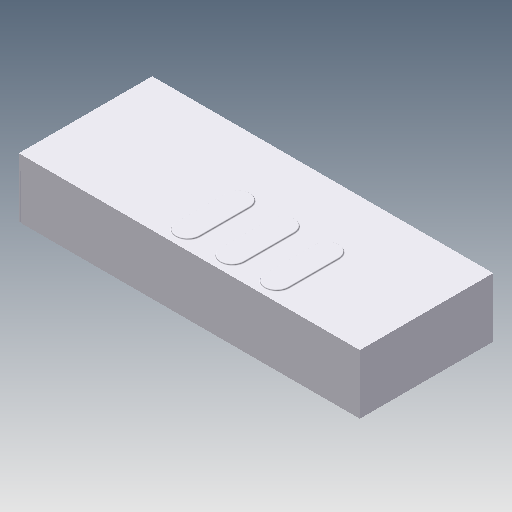
# Autodesk Inventor part: config - interface module
Saved by Autodesk Inventor 2020 (Build 240152000, 152)
## iProperties
Created: 2005-12-05
Part Number: config - interface module
Document SubType Name: Modeling
Designer: Simon.Ng@autodesk.com
Stock Number: config - interface module
Density: 1 g/cm^3
Material: Generic
Mass: 106.435 g
Surface Area: 212.581 cm^2
Volume: 106.435 cm^3
Appearance: Teflon
Company: Autodesk Asia Pte. Ltd.
Title: PC Demo
Author: Simon.Ng@autodesk.com
Autodesk Inventor part; units mm, degrees
ref_plane "YZ Plane" through (0, 0, 0) normal (1, 0, 0) x (0, 1, 0)
ref_plane "XZ Plane" through (0, 0, 0) normal (0, 1, 0) x (-1, 0, 0)
ref_plane "XY Plane" through (0, 0, 0) normal (0, 0, 1) x (1, 0, 0)
sketch "Sketch1" plane through (0, 0, 0) normal (0, 0, 1) x (1, 0, 0)
  line L0 (0, 26) -> (0, -2) projected
  line L1 (-69, 0) -> (92, 0) projected
  line L2 (-57.5, 0) -> (57.5, 0)
  line L3 (57.5, 0) -> (57.5, 20)
  line L4 (57.5, 20) -> (-57.5, 20)
  line L5 (-57.5, 20) -> (-57.5, 0)
  dimension "d0" = 115
  dimension "d1" = 20
  constraints: 8 end point, 2 parallel, 1 horizontal, 1 perpendicular, 1 point on line, 1 other
  measures "d0" distance of L3.end L4.end
  measures "d1" distance of L2.end L3.end
extrude "Extrusion1" add sketch "Sketch1" along normal blind 45
sketch "Sketch3" plane through (0, 0, 45) normal (0, 0, 1) x (1, 0, 0)
  line L0 (57.5, 0) -> (-57.5, 0) projected
  line L1 (57.5, 20) -> (57.5, 0) projected
  line L2 (57, 15) -> (56.8, 15)
  line L3 (56.8, 15) -> (56.8, 0)
  line L4 (56.8, 0) -> (57, 0)
  line L5 (57, 0) -> (57, 15)
  dimension "d8" = 0.5
  dimension "d9" = 0.2
  dimension "d10" = 15
  constraints: 8 end point, 2 parallel, 1 horizontal, 1 perpendicular, 1 point on line
  measures "d8" distance between parallel lines of L1 L5
  measures "d9" distance of L2.start L2.end
  measures "d10" distance of L2.end L3.end
extrude "Extrusion3" cut sketch "Sketch3" against normal blind 5
mirror "Mirror1" about plane through (0, 0, 0) normal (1, 0, 0) of "Extrusion3"
sketch "Sketch4" plane through (0, 0, 45) normal (0, 0, 1) x (1, 0, 0)
  line L0 (57.5, 20) -> (57.5, 0) construction
  line L1 (57, 15) -> (57.5, 15)
  constraints: 2 end point, 1 perpendicular, 1 point on line
split_face "Split1"
sketch "Sketch5" plane through (57.5, 0, 0) normal (1, 0, 0) x (0, 0, -1)
  line L0 (-45, 20) -> (-45, 15) construction
  line L1 (0, 20) -> (-45, 20) construction
  line L2 (-45, 15) -> (-25, 15)
  line L3 (-25, 15) -> (-15, 18)
  line L4 (-15, 18) -> (-15, 20)
  dimension "d13" = 30
  dimension "d14" = 2
  dimension "d15" = 20
  constraints: 6 end point, 1 parallel, 1 perpendicular, 1 point on line
  measures "d13" distance between parallel lines of L0 L4
  measures "d14" distance of L3.end L4.end
  measures "d15" distance of L0.end L2.end
split_face "Split2"
sketch "Sketch6" plane through (-57.5, 20, 0) normal (0, 1, 0) x (1, 0, 0)
  line L0 (0, -15) -> (0, -45) construction
  line L1 (115, -15) -> (0, -15)
  constraints: 2 end point, 1 perpendicular
split_face "Split3"
sketch "Sketch7" plane through (-57.5, 20, 45) normal (0, 1, 0) x (1, 0, 0)
  line L0 (0, 0) -> (115, 0) projected
  line L1 (115, 30) -> (115, 0) projected
  line L2 (77, 23) -> (85, 23)
  line L3 (85, 23) -> (85, 6)
  line L4 (85, 6) -> (77, 6)
  line L5 (77, 6) -> (77, 23)
  circle A0 centre (81, 23) radius 4
  circle A1 centre (81, 6) radius 4
  dimension "d16" = 25
  dimension "d17" = 8
  dimension "d18" = 30
  dimension "d19" = 6
  constraints: 8 end point, 2 horizontal alignment, 2 midpoint, 2 parallel, 1 horizontal, 1 perpendicular, 4 other
  measures "d17" distance between parallel lines of L5 L3
  measures "d18" distance between parallel lines of L1 L3
  measures "d19" distance between parallel lines of L0 L4
extrude "Extrusion4" add sketch "Sketch7" along normal blind 0.5
fillet "Fillet1" radius 0.25 8 edges at (23.5, 20, 43) (19.5, 20, 30.5) (23.5, 20, 18) (27.5, 20, 30.5) (23.5, 20.5, 43) (19.5, 20.5, 30.5) (23.5, 20.5, 18) (27.5, 20.5, 30.5)
pattern_linear "Rectangular Pattern1" count 3 spacing 15 along (-1, 0, 0) of "Extrusion4", "Fillet1"
sketch "Sketch8" plane through (-56.8, 0, 45) normal (0, -1, 0) x (1, 0, 0)
  line L0 (-0.7, -45) -> (114.3, -45) projected
  line L1 (114.3, -45) -> (114.3, 0) projected
  line L2 (0, -5) -> (-0.2, -5) projected
  line L3 (104.3, -10.1321) -> (104.3, -39.4486) construction
  line L4 (96.3, -15.2854) -> (96.3, -32.9211) construction
  circle A0 centre (104.3, -35) radius 3.5
  circle A1 centre (104.3, -35) radius 1.75
  circle A2 centre (104.3, -23) radius 3.5
  circle A3 centre (104.3, -23) radius 1.75
  circle A4 centre (104.3, -11) radius 3.5
  circle A5 centre (104.3, -11) radius 1.75
  circle A6 centre (96.3, -17) radius 1.75
  circle A7 centre (96.3, -17) radius 3.5
  circle A8 centre (96.3, -29) radius 1.75
  circle A9 centre (96.3, -29) radius 3.5
  dimension "d26" = 3.5
  dimension "d27" = 7
  dimension "d28" = 10
  dimension "d29" = 10
  dimension "d30" = 12
  dimension "d31" = 12
  dimension "d32" = 8
  dimension "d33" = 12
  dimension "d34" = 16
  constraints: 10 centre point, 8 equal radius, 5 coincident, 5 point on line, 4 end point, 1 parallel, 1 perpendicular
  measures "d26" diameter of A1
  measures "d27" diameter of A0
  measures "d28" distance between parallel lines of L1 L3
  measures "d29" distance from line of L0 A0.centre
  measures "d30" distance of A2.centre A0.centre
  measures "d31" distance of A2.centre A4.centre
  measures "d32" distance between parallel lines of L3 L4
  measures "d33" distance of A8.centre A6.centre
  measures "d34" distance from line of L0 A9.centre
extrude "Extrusion5" add sketch "Sketch8" along normal blind 5
sketch "Sketch9" plane through (-56.8, 0, 45) normal (0, -1, 0) x (1, 0, 0)
  line L0 (-0.7, -45) -> (114.3, -45) projected
  line L1 (114.3, -45) -> (114.3, 0) projected
  line L2 (0, -5) -> (-0.2, -5) projected
  circle A0 centre (79.3, -18) radius 6
  circle A1 centre (79.3, -33) radius 6
  line L3 (79.3, -18) -> (79.3, -33) construction
  dimension "d37" = 35
  dimension "d38" = 12
  dimension "d39" = 15
  dimension "d40" = 12
  constraints: 2 centre point, 2 end point, 1 equal radius, 1 perpendicular
  measures "d37" distance between parallel lines of L1 L3
  measures "d38" diameter of A1
  measures "d39" distance of L3.end L3.start
  measures "d40" distance from line of L0 L3.end
extrude "Extrusion6" add sketch "Sketch9" along normal blind 2
sketch "Sketch10" plane through (22.5, -2, 27) normal (0, -1, 0) x (1, 0, 0)
  circle A0 centre (0, 0) radius 6 projected
  line L0 (-4.0311, -2) -> (-2.5311, -2)
  line L1 (-2.5311, -2) -> (-2.5311, -3.7207)
  line L2 (4.0311, -2) -> (2.5311, -2)
  line L3 (2.5311, -2) -> (2.5311, -3.7207)
  line L4 (0, 0) -> (0, 4.5) construction
  line L5 (-1.5, 4.2426) -> (-1.5, 3.2426)
  line L6 (-1.5, 3.2426) -> (1.5, 3.2426)
  line L7 (1.5, 3.2426) -> (1.5, 4.2426)
  circle A1 centre (0, 0) radius 5
  arc A2 (-1.5, 4.2426) -> (-4.0311, -2) centre (0, 0) ccw
  arc A3 (-2.5311, -3.7207) -> (2.5311, -3.7207) centre (0, 0) ccw
  arc A4 (4.0311, -2) -> (1.5, 4.2426) centre (0, 0) ccw
  dimension "d44" = 2
  dimension "d45" = 1.5
  dimension "d46" = 3
  dimension "d47" = 1
  dimension "d48" = 10
  constraints: 16 end point, 6 point on circle, 4 centre point, 4 perpendicular, 3 parallel, 2 coincident, 2 equal length, 1 horizontal, 1 other
  measures "d44" distance from line of L0 A0.centre
  measures "d45" distance of L0.start L0.end
  measures "d46" distance of L5.end L6.end
  measures "d47" distance of L6.end L7.end
  measures "d48" diameter of A1
extrude "Extrusion7" cut sketch "Sketch10" against normal blind 5 contours A1
sketch "Sketch11" plane through (-56.8, -2, 45) normal (0, -1, 0) x (1, 0, 0)
  arc A0 (76.7689, -21.7207) -> (81.8311, -21.7207) centre (79.3, -18) ccw projected
  arc A1 (77.8, -13.7574) -> (75.2689, -20) centre (79.3, -18) ccw projected
  line L0 (75.2689, -20) -> (76.7689, -20) projected
  circle A2 centre (79.3, -18) radius 3 construction
  circle A3 centre (77.2604, -15.8) radius 0.25
  circle A4 centre (76.4716, -17) radius 0.25
  circle A5 centre (81.3396, -15.8) radius 0.25
  circle A6 centre (82.1284, -17) radius 0.25
  circle A7 centre (77.6417, -20.5) radius 0.25
  circle A8 centre (80.9583, -20.5) radius 0.25
  line L1 (79.3, -18) -> (79.3, -16.3241) construction
  line L2 (79, -15.5) -> (79.6, -15.5)
  line L3 (79.6, -15.5) -> (79.6, -17.5)
  line L4 (79.6, -17.5) -> (79, -17.5)
  line L5 (79, -17.5) -> (79, -15.5)
  dimension "d51" = 6
  dimension "d52" = 0.5
  dimension "d53" = 1
  dimension "d54" = 2.2
  dimension "d55" = 2.5
  dimension "d56" = 2
  dimension "d57" = 0.5
  dimension "d58" = 0.6
  constraints: 10 end point, 7 centre point, 6 point on circle, 5 equal radius, 3 symmetric about line, 2 parallel, 2 perpendicular, 1 coincident, 1 horizontal, 1 other
  measures "d51" diameter of A2
  measures "d52" diameter of A3
  measures "d53" vertical distance of A0.centre A4.centre
  measures "d54" vertical distance of A0.centre A3.centre
  measures "d55" vertical distance of A7.centre A0.centre
  measures "d56" distance of L4.end L2.start
  measures "d57" distance from line of A0.centre L4
  measures "d58" distance of L2.start L2.end
extrude "Extrusion8" cut sketch "Sketch11" against normal blind 3
pattern_linear "Rectangular Pattern2" count 2 spacing 15 along (0, 0, -1) of "Extrusion7", "Extrusion8"
sketch "Sketch12" plane through (-56.8, 0, 45) normal (0, -1, 0) x (1, 0, 0)
  line L0 (-0.7, -45) -> (-0.7, 0) projected
  line L1 (-0.7, -45) -> (114.3, -45) projected
  line L2 (113.6, 0) -> (0, 0) projected
  line L3 (0, -5) -> (-0.2, -5) projected
  line L4 (46.3, -28) -> (63.3, -28)
  line L5 (63.3, -28) -> (61.3, -35)
  line L6 (61.3, -35) -> (48.3, -35)
  line L7 (48.3, -35) -> (46.3, -28)
  line L8 (14.3, -28) -> (31.3, -28)
  line L9 (31.3, -28) -> (29.3, -35)
  line L10 (29.3, -35) -> (16.3, -35)
  line L11 (16.3, -35) -> (14.3, -28)
  line L12 (21.3, -12) -> (53.3, -12)
  line L13 (53.3, -12) -> (51.3, -20)
  line L14 (51.3, -20) -> (23.3, -20)
  line L15 (23.3, -20) -> (21.3, -12)
  dimension "d64" = 7
  dimension "d65" = 17
  dimension "d66" = 13
  dimension "d67" = 32
  dimension "d68" = 28
  dimension "d69" = 10
  dimension "d70" = 15
  dimension "d71" = 15
  dimension "d72" = 12
  dimension "d73" = 8
  dimension "d74" = 22
  constraints: 24 end point, 8 parallel, 3 equal length, 2 collinear
  measures "d64" distance between parallel lines of L10 L8
  measures "d65" distance of L8.start L8.end
  measures "d66" distance of L9.end L10.end
  measures "d67" distance of L12.start L12.end
  measures "d68" distance of L13.end L14.end
  measures "d69" distance between parallel lines of L1 L10
  measures "d70" distance from line of L0 L8.start
  measures "d71" distance of L4.start L8.end
  measures "d72" distance between parallel lines of L12 L2
  measures "d73" distance between parallel lines of L12 L14
  measures "d74" distance from line of L0 L12.start
extrude "Extrusion9" add sketch "Sketch12" along normal blind 5
fillet "Fillet2" radius 1 6 edges at (-35.5, -2.5, 33) (-3.5, -2.5, 33) (-42.5, -2.5, 17) (-25.5, -2.5, 17) (-10.5, -2.5, 17) (6.5, -2.5, 17)
fillet "Fillet2" radius 1 6 edges at (-33.5, -2.5, 25) (-5.5, -2.5, 25) (-40.5, -2.5, 10) (-27.5, -2.5, 10) (-8.5, -2.5, 10) (4.5, -2.5, 10)
sketch "Sketch16" plane through (-56.8, -5, 45) normal (0, -1, 0) x (1, 0, 0)
  line L0 (47.6257, -28) -> (61.9743, -28) construction
  line L1 (60.5457, -35) -> (49.0543, -35) construction
  line L2 (54.8, -28) -> (54.8, -35) construction
  line L3 (54.8, -31.5) -> (57.6719, -31.5) construction
  line L4 (54.8, -29.75) -> (60.918, -29.75) construction
  circle A0 centre (55.3, -31.5) radius 0.5
  circle A1 centre (57.8, -31.5) radius 0.5
  circle A2 centre (60.3, -31.5) radius 0.5
  line L5 (54.8, -31.5) -> (46.0208, -31.5) construction
  circle A3 centre (52.8, -31.5) radius 0.5
  circle A4 centre (50.3, -31.5) radius 0.5
  line L6 (57.8, -31.5) -> (59.05, -29.75) construction
  line L7 (60.3, -31.5) -> (59.05, -29.75) construction
  circle A5 centre (59.05, -29.75) radius 0.5
  circle A6 centre (56.55, -29.75) radius 0.5
  circle A7 centre (54.05, -29.75) radius 0.5
  circle A8 centre (51.55, -29.75) radius 0.5
  circle A9 centre (49.05, -29.75) radius 0.5
  circle A10 centre (59.05, -33.25) radius 0.5
  circle A11 centre (56.55, -33.25) radius 0.5
  circle A12 centre (54.05, -33.25) radius 0.5
  circle A13 centre (51.55, -33.25) radius 0.5
  circle A14 centre (49.05, -33.25) radius 0.5
  point P0 (54.8, -33.25)
  dimension "d85" = 1.75
  dimension "d86" = 1
  dimension "d87" = 2.5
  dimension "d88" = 2.5
  dimension "d89" = 2.5
  dimension "d90" = 2.5
  dimension "d91" = 2
  dimension "d92" = 2.5
  dimension "d93" = 2.5
  dimension "d94" = 2.5
  dimension "d95" = 2.5
  constraints: 15 centre point, 12 end point, 11 point on line, 9 equal radius, 7 symmetric about line, 3 midpoint, 2 coincident, 2 parallel, 1 equal length, 1 perpendicular, 5 other
  measures "d85" distance between parallel lines of L4 L0
  measures "d86" diameter of A4
  measures "d87" distance of A3.centre A4.centre
  measures "d88" distance of A0.centre A3.centre
  measures "d89" distance of L6.start A0.centre
  measures "d90" distance of L7.start L6.start
  measures "d91" distance from line of L2 A3.centre
  measures "d92" distance of L6.end A6.centre
  measures "d93" distance of A6.centre A7.centre
  measures "d94" distance of A7.centre A8.centre
  measures "d95" distance of A8.centre A9.centre
extrude "Extrusion11" cut sketch "Sketch16" against normal blind 5
sketch "Sketch17" plane through (-56.8, -5, 45) normal (0, -1, 0) x (1, 0, 0)
  arc A0 (28.5457, -35) -> (29.5072, -34.2747) centre (28.5457, -34) ccw projected
  line L0 (30.9358, -29.2747) -> (29.5072, -34.2747) projected
  arc A1 (30.9358, -29.2747) -> (29.9743, -28) centre (29.9743, -29) ccw projected
  line L1 (15.6257, -28) -> (29.9743, -28) projected
  arc A2 (15.6257, -28) -> (14.6642, -29.2747) centre (15.6257, -29) ccw projected
  line L2 (16.0928, -34.2747) -> (14.6642, -29.2747) projected
  arc A3 (16.0928, -34.2747) -> (17.0543, -35) centre (17.0543, -34) ccw projected
  line L3 (28.5457, -35) -> (17.0543, -35) projected
  line L4 (22.8, -28) -> (22.8, -35) construction
  line L5 (22.8, -31.5) -> (25.7779, -31.5) construction
  line L6 (17.5672, -29.75) -> (27.661, -29.75) construction
  line L7 (22.8, -31.5) -> (14.4431, -31.5) construction
  circle A4 centre (23.3, -31.5) radius 0.5
  circle A5 centre (20.8, -31.5) radius 0.5
  circle A6 centre (18.3, -31.5) radius 0.5
  circle A7 centre (25.8, -31.5) radius 0.5
  circle A8 centre (28.3, -31.5) radius 0.5
  line L8 (25.8, -31.5) -> (27.05, -29.75) construction
  line L9 (28.3, -31.5) -> (27.05, -29.75) construction
  circle A9 centre (27.05, -29.75) radius 0.5
  circle A10 centre (24.55, -29.75) radius 0.5
  circle A11 centre (22.05, -29.75) radius 0.5
  circle A12 centre (19.55, -29.75) radius 0.5
  circle A13 centre (17.05, -29.75) radius 0.5
  line L10 (17.5672, -33.25) -> (27.661, -33.25) construction
  circle A14 centre (27.05, -33.25) radius 0.5
  circle A15 centre (24.55, -33.25) radius 0.5
  circle A16 centre (22.05, -33.25) radius 0.5
  circle A17 centre (19.55, -33.25) radius 0.5
  circle A18 centre (17.05, -33.25) radius 0.5
  arc A19 (30.455, -29.1374) -> (29.9743, -28.5) centre (29.9743, -29) ccw
  line L11 (30.455, -29.1374) -> (29.0265, -34.1374)
  arc A20 (28.5457, -34.5) -> (29.0265, -34.1374) centre (28.5457, -34) ccw
  line L12 (28.5457, -34.5) -> (17.0543, -34.5)
  arc A21 (16.5735, -34.1374) -> (17.0543, -34.5) centre (17.0543, -34) ccw
  line L13 (16.5735, -34.1374) -> (15.145, -29.1374)
  arc A22 (15.6257, -28.5) -> (15.145, -29.1374) centre (15.6257, -29) ccw
  line L14 (15.6257, -28.5) -> (29.9743, -28.5)
  dimension "d98" = 1.75
  dimension "d99" = 2.5
  dimension "d100" = 2.5
  dimension "d101" = 2.5
  dimension "d102" = 2.5
  dimension "d103" = 2
  dimension "d104" = 1
  dimension "d105" = 2.5
  dimension "d106" = 2.5
  dimension "d107" = 2.5
  dimension "d108" = 2.5
  dimension "d109" = 0.5
  constraints: 22 end point, 19 centre point, 15 point on line, 9 equal radius, 8 point on circle, 8 symmetric about line, 3 midpoint, 2 coincident, 2 parallel, 1 equal length, 1 perpendicular, 12 other
  measures "d98" distance between parallel lines of L6 L1
  measures "d99" distance of A5.centre A6.centre
  measures "d100" distance of A4.centre A5.centre
  measures "d101" distance of L8.start A4.centre
  measures "d102" distance of L9.start L8.start
  measures "d103" distance from line of L4 A5.centre
  measures "d104" diameter of A6
  measures "d105" distance of L8.end A10.centre
  measures "d106" distance of A10.centre A11.centre
  measures "d107" distance of A11.centre A12.centre
  measures "d108" distance of A12.centre A13.centre
  measures "d109" distance between parallel lines of L1 L14
extrude "Extrusion12" cut sketch "Sketch17" against normal blind 5 contours L11 A20 L12 A21 L13 A22 L14 A19
fillet "Fillet3" radius 0.5 15 edges at (-40.25, -5, 15.25) (-37.75, -5, 15.25) (-35.25, -5, 15.25) (-32.75, -5, 15.25) (-30.25, -5, 15.25) (-29, -5, 13.5) (-31.5, -5, 13.5) (-34, -5, 13.5) (-36.5, -5, 13.5) (-39, -5, 13.5) (-40.25, -5, 11.75) (-37.75, -5, 11.75) (-35.25, -5, 11.75) (-32.75, -5, 11.75) (-30.25, -5, 11.75)
sketch "Sketch18" plane through (-56.8, -5, 45) normal (0, -1, 0) x (1, 0, 0)
  line L0 (22.5808, -12) -> (52.0192, -12) projected
  line L1 (50.5192, -20) -> (24.0808, -20) projected
  line L2 (37.3, -12) -> (37.3, -20) construction
  line L3 (24.1, -14.6667) -> (50.5, -14.6667) construction
  line L4 (25.2, -17.3333) -> (49.4, -17.3333) construction
  circle A0 centre (37.3, -14.6667) radius 0.75
  circle A1 centre (35.1, -14.6667) radius 0.75
  circle A2 centre (32.9, -14.6667) radius 0.75
  circle A3 centre (30.7, -14.6667) radius 0.75
  circle A4 centre (28.5, -14.6667) radius 0.75
  circle A5 centre (26.3, -14.6667) radius 0.75
  circle A6 centre (24.1, -14.6667) radius 0.75
  circle A7 centre (39.5, -14.6667) radius 0.75
  circle A8 centre (41.7, -14.6667) radius 0.75
  circle A9 centre (43.9, -14.6667) radius 0.75
  circle A10 centre (46.1, -14.6667) radius 0.75
  circle A11 centre (48.3, -14.6667) radius 0.75
  circle A12 centre (50.5, -14.6667) radius 0.75
  line L5 (24.1, -14.6667) -> (25.2, -17.3333) construction
  line L6 (26.3, -14.6667) -> (25.2, -17.3333) construction
  circle A13 centre (25.2, -17.3333) radius 0.75
  circle A14 centre (27.4, -17.3333) radius 0.75
  circle A15 centre (29.6, -17.3333) radius 0.75
  circle A16 centre (31.8, -17.3333) radius 0.75
  circle A17 centre (34, -17.3333) radius 0.75
  circle A18 centre (36.2, -17.3333) radius 0.75
  circle A19 centre (38.4, -17.3333) radius 0.75
  circle A20 centre (40.6, -17.3333) radius 0.75
  circle A21 centre (42.8, -17.3333) radius 0.75
  circle A22 centre (45, -17.3333) radius 0.75
  circle A23 centre (47.2, -17.3333) radius 0.75
  circle A24 centre (49.4, -17.3333) radius 0.75
  dimension "d114" = 2.6667
  dimension "d113" = 2.6667
  dimension "d115" = 2.2
  dimension "d116" = 2.2
  dimension "d117" = 2.2
  dimension "d118" = 2.2
  dimension "d119" = 2.2
  dimension "d120" = 2.2
  dimension "d121" = 1.5
  dimension "d122" = 2.2
  dimension "d123" = 2.2
  dimension "d124" = 2.2
  dimension "d125" = 2.2
  dimension "d126" = 2.2
  dimension "d127" = 2.2
  dimension "d128" = 2.2
  dimension "d129" = 2.2
  dimension "d130" = 2.2
  dimension "d131" = 2.2
  constraints: 25 centre point, 24 equal radius, 8 symmetric about line, 6 end point, 4 coincident, 2 midpoint, 1 equal length, 1 point on line, 1 vertical, 27 other
  measures "d115" distance of A0.centre A1.centre
  measures "d116" distance of A1.centre A2.centre
  measures "d117" distance of A2.centre A3.centre
  measures "d118" distance of A3.centre A4.centre
  measures "d119" distance of A4.centre L6.start
  measures "d120" distance of L6.start point (24.1, -14.667)
  measures "d121" diameter of A6
  measures "d122" distance of A14.centre L5.end
  measures "d123" distance of A15.centre A14.centre
  measures "d124" distance of A16.centre A15.centre
  measures "d125" distance of A17.centre A16.centre
  measures "d126" distance of A18.centre A17.centre
  measures "d127" distance of A19.centre A18.centre
  measures "d128" distance of A20.centre A19.centre
  measures "d129" distance of A21.centre A20.centre
  measures "d130" distance of A22.centre A21.centre
  measures "d131" distance of A23.centre A22.centre
extrude "Extrusion13" cut sketch "Sketch18" against normal blind 5
sketch "Sketch19" plane through (-56.8, 0, 45) normal (0, -1, 0) x (1, 0, 0)
  line L0 (62.9358, -29.2747) -> (61.5072, -34.2747) projected
  line L1 (48.0928, -34.2747) -> (46.6642, -29.2747) projected
  line L2 (30.9358, -29.2747) -> (29.5072, -34.2747) projected
  line L3 (16.0928, -34.2747) -> (14.6642, -29.2747) projected
  line L4 (15.6257, -28) -> (29.9743, -28) projected
  line L5 (52.9894, -13.2425) -> (51.4894, -19.2425) projected
  line L6 (23.1106, -19.2425) -> (21.6106, -13.2425) projected
  line L7 (22.5808, -12) -> (52.0192, -12) projected
  line L8 (113.6, 0) -> (0, 0) projected
  line L9 (7.3411, -32) -> (68.4391, -32) construction
  line L10 (14.219, -16) -> (57.884, -16) construction
  line L11 (12.3896, -30.5009) -> (13.7144, -31.2043)
  line L12 (13.7144, -31.2043) -> (13.7677, -32.7034)
  line L13 (13.7677, -32.7034) -> (12.4961, -33.4991)
  line L14 (12.4961, -33.4991) -> (11.1713, -32.7957)
  line L15 (11.1713, -32.7957) -> (11.118, -31.2966)
  line L16 (11.118, -31.2966) -> (12.3896, -30.5009)
  line L17 (33.6228, -30.5741) -> (34.6248, -31.6903)
  line L18 (34.6248, -31.6903) -> (34.1592, -33.1162)
  line L19 (34.1592, -33.1162) -> (32.6915, -33.4259)
  line L20 (32.6915, -33.4259) -> (31.6895, -32.3097)
  line L21 (31.6895, -32.3097) -> (32.1551, -30.8838)
  line L22 (32.1551, -30.8838) -> (33.6228, -30.5741)
  line L23 (43.2748, -31.059) -> (44.6738, -30.5179)
  line L24 (44.6738, -30.5179) -> (45.8419, -31.4589)
  line L25 (45.8419, -31.4589) -> (45.611, -32.941)
  line L26 (45.611, -32.941) -> (44.212, -33.4821)
  line L27 (44.212, -33.4821) -> (43.0439, -32.5411)
  line L28 (43.0439, -32.5411) -> (43.2748, -31.059)
  line L29 (65.1617, -30.5) -> (66.4584, -31.2539)
  line L30 (66.4584, -31.2539) -> (66.4539, -32.7539)
  line L31 (66.4539, -32.7539) -> (65.1526, -33.5)
  line L32 (65.1526, -33.5) -> (63.8559, -32.7461)
  line L33 (63.8559, -32.7461) -> (63.8604, -31.2461)
  line L34 (63.8604, -31.2461) -> (65.1617, -30.5)
  line L35 (19.7505, -17.4308) -> (18.2862, -17.1055)
  line L36 (18.2862, -17.1055) -> (17.8357, -15.6748)
  line L37 (17.8357, -15.6748) -> (18.8495, -14.5692)
  line L38 (18.8495, -14.5692) -> (20.3138, -14.8945)
  line L39 (20.3138, -14.8945) -> (20.7643, -16.3252)
  line L40 (20.7643, -16.3252) -> (19.7505, -17.4308)
  line L41 (56.5613, -16.8119) -> (55.2276, -17.4982)
  line L42 (55.2276, -17.4982) -> (53.9663, -16.6864)
  line L43 (53.9663, -16.6864) -> (54.0387, -15.1881)
  line L44 (54.0387, -15.1881) -> (55.3724, -14.5018)
  line L45 (55.3724, -14.5018) -> (56.6337, -15.3136)
  line L46 (56.6337, -15.3136) -> (56.5613, -16.8119)
  point P0 (12.4429, -32)
  point P1 (33.1571, -32)
  point P2 (44.4429, -32)
  point P3 (65.1571, -32)
  point P4 (19.3, -16)
  point P5 (55.3, -16)
  point P6 (15.4429, -32)
  point P7 (30.1571, -32)
  point P8 (47.4429, -32)
  point P9 (62.1571, -32)
  point P10 (22.3, -16)
  point P11 (52.3, -16)
  dimension "d134" = 4
  dimension "d135" = 4
  dimension "d136" = 1.5
  dimension "d137" = 3
  dimension "d138" = 3
  dimension "d139" = 3
  dimension "d140" = 3
  dimension "d141" = 3
  dimension "d142" = 3
  constraints: 74 end point, 10 point on line, 5 equal length, 2 horizontal, 77 other
  measures "d135" distance between parallel lines of L10 L7
  measures "d136" distance of L15.end L11.start
  measures "d137" distance of point (15.443, -32) point (12.443, -32)
  measures "d138" distance of point (33.157, -32) point (30.157, -32)
  measures "d139" distance of point (47.443, -32) point (44.443, -32)
  measures "d140" distance of point (62.157, -32) point (65.157, -32)
  measures "d141" distance of point (55.3, -16) point (52.3, -16)
  measures "d142" distance of point (22.3, -16) point (19.3, -16)
extrude "Extrusion14" add sketch "Sketch19" along normal blind 5.5
sketch "Sketch20" plane through (-56.8, -5.5, 45) normal (0, -1, 0) x (1, 0, 0)
  line L0 (18.2862, -17.1055) -> (17.8357, -15.6748) construction
  line L1 (20.3138, -14.8945) -> (20.7643, -16.3252) construction
  line L2 (13.7144, -31.2043) -> (13.7677, -32.7034) construction
  line L3 (12.3896, -30.5009) -> (13.7144, -31.2043) construction
  line L4 (11.118, -31.2966) -> (12.3896, -30.5009) construction
  line L5 (11.1713, -32.7957) -> (11.118, -31.2966) construction
  line L6 (12.4961, -33.4991) -> (11.1713, -32.7957) construction
  line L7 (13.7677, -32.7034) -> (12.4961, -33.4991) construction
  line L8 (34.6248, -31.6903) -> (34.1592, -33.1162) construction
  line L9 (33.6228, -30.5741) -> (34.6248, -31.6903) construction
  line L10 (32.1551, -30.8838) -> (33.6228, -30.5741) construction
  line L11 (31.6895, -32.3097) -> (32.1551, -30.8838) construction
  line L12 (32.6915, -33.4259) -> (31.6895, -32.3097) construction
  line L13 (34.1592, -33.1162) -> (32.6915, -33.4259) construction
  line L14 (44.6738, -30.5179) -> (45.8419, -31.4589) construction
  line L15 (43.2748, -31.059) -> (44.6738, -30.5179) construction
  line L16 (43.0439, -32.5411) -> (43.2748, -31.059) construction
  line L17 (44.212, -33.4821) -> (43.0439, -32.5411) construction
  line L18 (45.611, -32.941) -> (44.212, -33.4821) construction
  line L19 (45.8419, -31.4589) -> (45.611, -32.941) construction
  line L20 (55.2276, -17.4982) -> (53.9663, -16.6864) construction
  line L21 (56.5613, -16.8119) -> (55.2276, -17.4982) construction
  line L22 (56.6337, -15.3136) -> (56.5613, -16.8119) construction
  line L23 (55.3724, -14.5018) -> (56.6337, -15.3136) construction
  line L24 (54.0387, -15.1881) -> (55.3724, -14.5018) construction
  line L25 (53.9663, -16.6864) -> (54.0387, -15.1881) construction
  line L26 (66.4584, -31.2539) -> (66.4539, -32.7539) construction
  line L27 (65.1617, -30.5) -> (66.4584, -31.2539) construction
  line L28 (63.8604, -31.2461) -> (65.1617, -30.5) construction
  line L29 (63.8559, -32.7461) -> (63.8604, -31.2461) construction
  line L30 (65.1526, -33.5) -> (63.8559, -32.7461) construction
  line L31 (66.4539, -32.7539) -> (65.1526, -33.5) construction
  line L32 (18.8495, -14.5692) -> (19.7505, -17.4308) construction
  line L33 (18.0609, -16.3901) -> (20.5391, -15.6099) construction
  line L34 (55.3724, -14.5018) -> (55.2276, -17.4982) construction
  line L35 (54.0025, -15.9373) -> (56.5975, -16.0627) construction
  line L36 (12.3896, -30.5009) -> (12.4961, -33.4991) construction
  line L37 (11.1446, -32.0461) -> (13.7411, -31.9539) construction
  line L38 (33.6228, -30.5741) -> (32.6915, -33.4259) construction
  line L39 (31.9223, -31.5968) -> (34.392, -32.4032) construction
  line L40 (44.6738, -30.5179) -> (44.212, -33.4821) construction
  line L41 (43.1593, -31.8) -> (45.7264, -32.2) construction
  line L42 (65.1617, -30.5) -> (65.1526, -33.5) construction
  line L43 (63.8581, -31.9961) -> (66.4562, -32.0039) construction
  point P0 (65.1571, -32)
  point P1 (55.3, -16)
  point P2 (44.4429, -32)
  point P3 (33.1571, -32)
  point P4 (19.3, -16)
  point P5 (12.4429, -32)
  constraints: 24 end point, 18 midpoint, 5 parallel
hole "Hole1" at (8.3571, -5.5, 13) at (-1.5, -5.5, 29) at (-12.3571, -5.5, 13) at (-23.6429, -5.5, 13) at (-37.5, -5.5, 29) at (-44.3571, -5.5, 13) direction (0, 1, 0) diameter 1.583 depth 4 thread size "M1.8x0.2" class "6H" standard "ISO Metric profile"
equation "\"d88\" = d87"
equation "\"d89\" = d88"
equation "\"d90\" = d89"
equation "\"d92\" = d90"
equation "\"d93\" = d92"
equation "\"d94\" = d93"
equation "\"d95\" = d94"
equation "\"d100\" = d99"
equation "\"d101\" = d100"
equation "\"d102\" = d101"
equation "\"d105\" = d102"
equation "\"d106\" = d105"
equation "\"d107\" = d106"
equation "\"d108\" = d107"
equation "\"d114\" = d113"
equation "\"d116\" = d115"
equation "\"d117\" = d116"
equation "\"d118\" = d117"
equation "\"d119\" = d118"
equation "\"d120\" = d119"
equation "\"d122\" = d119"
equation "\"d123\" = d122"
equation "\"d124\" = d123"
equation "\"d125\" = d124"
equation "\"d126\" = d125"
equation "\"d127\" = d126"
equation "\"d128\" = d127"
equation "\"d129\" = d128"
equation "\"d130\" = d128"
equation "\"d131\" = d128"
equation "\"d138\" = d137"
equation "\"d139\" = d138"
equation "\"d140\" = d139"
equation "\"d141\" = d140"
equation "\"d142\" = d137"
body "Solid1"
